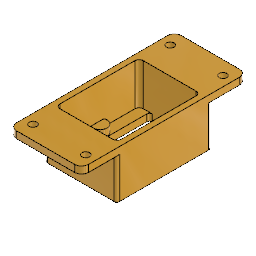
new_power_switch v3 (Autodesk Fusion 360 design; units mm, degrees)
Autodesk Fusion 360 part; units mm, degrees
sketch "Sketch1" plane through (0, 0, 0) normal (0, 0, 1) x (1, 0, 0)
  line L0 (26, -59.4) -> (-26, -59.4)
  line L1 (-26, -59.4) -> (-26, 59.4)
  line L2 (-26, 59.4) -> (26, 59.4)
  line L3 (26, 59.4) -> (26, -59.4)
  line L4 (26, -59.4) -> (-26, 59.4) construction
  line L5 (-26, -59.4) -> (26, 59.4) construction
  line L6 (14.5, -30) -> (-14.5, -30)
  line L7 (-14.5, -30) -> (-14.5, 30)
  line L8 (-14.5, 30) -> (14.5, 30)
  line L9 (14.5, 30) -> (14.5, -30)
  line L10 (14.5, -30) -> (-14.5, 30) construction
  line L11 (-14.5, -30) -> (14.5, 30) construction
  circle A0 centre (20, 0) radius 2.55
  circle A1 centre (-20, 0) radius 2.55
  line L12 (0, 0) -> (20, 0)
  line L13 (-20, 0) -> (0, 0)
  line L14 (26, -49.4) -> (-26, -49.4) construction
  line L15 (-26, -49.4) -> (-26, 49.4) construction
  line L16 (-26, 49.4) -> (26, 49.4) construction
  line L17 (26, 49.4) -> (26, -49.4) construction
  line L18 (26, -49.4) -> (-26, 49.4) construction
  line L19 (-26, -49.4) -> (26, 49.4) construction
  circle A2 centre (19, 49.4) radius 2.7
  circle A3 centre (-19, 49.4) radius 2.7
  circle A4 centre (-19, -49.4) radius 2.7
  circle A5 centre (19, -49.4) radius 2.7
  line L20 (22, -30) -> (-22, -30)
  line L21 (-22, -30) -> (-22, 30)
  line L22 (-22, 30) -> (22, 30)
  line L23 (22, 30) -> (22, -30)
  line L24 (22, -30) -> (-22, 30) construction
  line L25 (-22, -30) -> (22, 30) construction
  line L26 (26, -34) -> (-26, -34)
  line L27 (-26, -34) -> (-26, 34)
  line L28 (-26, 34) -> (26, 34)
  line L29 (26, 34) -> (26, -34)
  line L30 (26, -34) -> (-26, 34) construction
  line L31 (-26, -34) -> (26, 34) construction
  circle A6 centre (20, 0) radius 5
  circle A7 centre (-20, 0) radius 5
  dimension "d1" = 118.8
  dimension "d2" = 52
  dimension "d3" = 40
  dimension "d4" = 98.8
  dimension "d5" = 29
  dimension "d6" = 60
  dimension "d7" = 5.1
  dimension "d8" = 5.1
  dimension "d9" = 5.4
  dimension "d10" = 7
  dimension "d11" = 5.4
  dimension "d12" = 7
  dimension "d13" = 5.4
  dimension "d14" = 7
  dimension "d15" = 5.4
  dimension "d16" = 7
  dimension "d25" = 68
  dimension "d33" = 4
  dimension "d34" = 4
  dimension "d39" = 10
  dimension "d40" = 10
  constraint perpendicular L0 L1
  constraint parallel L0 L2
  constraint parallel L1 L3
  constraint horizontal L0
  constraint coincident L4 L12.start
  constraint coincident L5 L12.start
  constraint coincident L12.start L13.end
  constraint perpendicular L6 L7
  constraint parallel L6 L8
  constraint parallel L7 L9
  constraint horizontal L6
  constraint coincident L10 L12.start
  constraint coincident L11 L12.start
  constraint coincident A0.centre L12.end
  constraint perpendicular L9 L12
  constraint coincident A1.centre L13.start
  constraint parallel L12 L13
  constraint equal L12 L13
  constraint perpendicular L14 L15
  constraint parallel L14 L16
  constraint parallel L15 L17
  constraint horizontal L14
  constraint coincident L3 L14.start
  constraint coincident L18 L12.start
  constraint coincident L19 L12.start
  constraint coincident L16 A2.centre
  constraint coincident L16 A3.centre
  constraint coincident L14 A4.centre
  constraint coincident L14 A5.centre
  constraint perpendicular L20 L21
  constraint parallel L20 L22
  constraint parallel L21 L23
  constraint horizontal L20
  constraint coincident L24 L12.start
  constraint coincident L25 L12.start
  constraint perpendicular L26 L27
  constraint parallel L26 L28
  constraint parallel L27 L29
  constraint horizontal L26
  constraint coincident L3 L26.start
  constraint coincident L30 L12.start
  constraint coincident L31 L12.start
  constraint concentric A0 A6
  constraint concentric A1 A7
  measures "d1" distance of L0.end L1.end
  measures "d2" distance of L1.end L2.end
  measures "d3" distance of A0.centre A1.centre
  measures "d4" distance of L14 L16
  measures "d5" distance of L6.start L6.end
  measures "d6" distance of L6.end L7.end
  measures "d7" diameter of A1
  measures "d8" diameter of A0
  measures "d9" diameter of A2
  measures "d10" distance of L3 A2.centre
  measures "d11" diameter of A3
  measures "d12" distance of L1 A3.centre
  measures "d13" diameter of A4
  measures "d14" distance of L15 A4.centre
  measures "d15" diameter of A5
  measures "d16" distance of L3 A5.centre
  measures "d25" distance of L26 L28
  measures "d33" distance of L20 L26
  measures "d34" distance of L3 L23
  measures "d39" diameter of A6
  measures "d40" diameter of A7
extrude "Extrude4" add sketch "Sketch1" along normal blind 5 from surface at 30 contours L0 L1 L3 L26 | L1 L2 L3 L28 makes body 1 at (-5.7722, -38.4297, 30) makes body 2 at (-5.7722, 38.4297, 30)
extrude "Extrude5" add sketch "Sketch1" along normal up to surface (35 mm away) contours L1 L3 L26 L27 L28 L29 | A0 L23 A6 | A1 L21 A7 | A0 L23 | A1 L21 picked at (22.1757, -0.1134) picked at (-22.1623, 0.188) bodies 2 1
extrude "Extrude6" add sketch "Sketch1" along normal blind 5 contours L9 L12 L20 L23 A6 | L7 L13 L20 L21 A7 | L9 L12 L22 L23 A6 | L7 L13 L21 L22 A7 | A0 L12 L23 A6 | A0 L12 L23 A6 | A1 L13 L21 A7 | A1 L13 L21 A7 | A0 L23 | A1 L21 picked at (20.3521, 0.2438) picked at (-20.3254, 0.1232) bodies 2
extrude "Extrude7" add sketch "Sketch1" along normal blind 10 contours A0 L12 L23 A6 | A0 L12 L23 A6 | A0 L23 A6 | A1 L13 L21 A7 | A1 L13 L21 A7 | A1 L21 A7 | A0 L23 | A0 L23 | A1 L21 | A1 L21 bodies 2
extrude "Extrude8" cut sketch "Sketch1" along normal blind 8 contours A0 L23 | A0 L23 | A1 L21 | A1 L21 bodies 2
sketch "Sketch4" plane through (0, 0, 30) normal (0, 0, -1) x (1, 0, 0)
  line L0 (-26, -59.4) -> (26, -59.4)
  line L1 (26, -59.4) -> (26, -34)
  line L2 (26, -34) -> (-26, -34)
  line L3 (-26, -34) -> (-26, -59.4)
  circle A0 centre (19, -49.4) radius 2.7
  circle A1 centre (-19, -49.4) radius 2.7
  circle A2 centre (-19, 49.4) radius 2.7
  circle A3 centre (19, 49.4) radius 2.7
extrude "Extrude12" add sketch "Sketch4" against normal blind 0.2 contours A0 | A1 | A2 | A3 bodies 2
fillet "Fillet2" radius 2 4 edges at (-26, 34, 15) (26, 34, 15) (-26, -34, 15) (26, -34, 15) on bodies 2
fillet "Fillet1" radius 5 4 edges at (-26, -59.4, 32.5) (26, -59.4, 32.5) (26, 59.4, 32.5) (-26, 59.4, 32.5) on bodies 2
chamfer "Chamfer1" distance 0.6 angle 45 8 edges at (-25.4142, 33.4142, 0) (0, 34, 0) (25.4142, 33.4142, 0) (26, 0, 0) (25.4142, -33.4142, 0) (0, -34, 0) (-25.4142, -33.4142, 0) (-26, 0, 0) on bodies 2
fillet "Fillet3" radius 3 4 edges at (22, 30, 20) (-22, 30, 20) (-22, -30, 20) (22, -30, 20) on bodies 2
fillet "Fillet4" radius 2 4 edges at (-14.5, 30, 2.5) (14.5, 30, 2.5) (-14.5, -30, 2.5) (14.5, -30, 2.5) on bodies 2
equation "d1 = 68.8 mm + 60 mm - 10 mm"
equation "d4 = 68.8 mm + 30 mm"
equation "d7 = d8"
equation "d11 = d9"
equation "d13 = d9"
equation "d14 = d10"
equation "d15 = d9"
equation "d16 = d10"
equation "d40 = d39"
